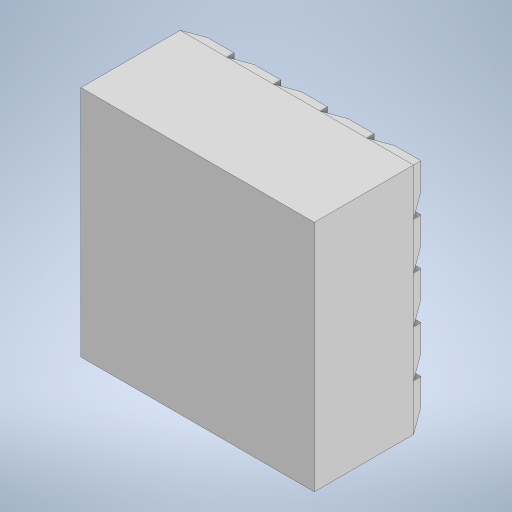
# Autodesk Inventor part: LI0013-FOOT
Saved by Autodesk Inventor 2023 (Build 270158000, 158)
## iProperties
Created: 2023-05-02
Part Number: LI0013-FOOT
Material: Generic
Document SubType Name: Modeling
Designer: Louis
Density: 1 g/cm^3
Appearance: Default
Author: Louis
Autodesk Inventor part; units mm, degrees
ref_plane "YZ Plane" through (0, 0, 0) normal (1, 0, 0) x (0, 1, 0)
ref_plane "XZ Plane" through (0, 0, 0) normal (0, 1, 0) x (-1, 0, 0)
ref_plane "XY Plane" through (0, 0, 0) normal (0, 0, 1) x (1, 0, 0)
sketch "Sketch1" plane through (0, 0, 0) normal (0, 0, 1) x (1, 0, 0)
  line L0 (-20, 20) -> (20, 20)
  line L1 (20, 20) -> (20, -20)
  line L2 (20, -20) -> (-20, -20)
  line L3 (-20, -20) -> (-20, 20)
  point P0 (0, 0)
  point P1 (-20, 0)
  point P2 (0, 20)
  dimension "d0" = 40
  dimension "d1" = 40
  constraints: 8 end point, 2 midpoint, 2 parallel, 1 horizontal, 1 horizontal alignment, 1 perpendicular, 1 vertical alignment
  measures "d0" distance of L0.start L0.end
  measures "d1" distance of L0.end L1.end
extrude "Extrusion1" add sketch "Sketch1" along normal blind 20
sketch "Sketch2" plane through (-20, -20, 0) normal (0, -1, 0) x (1, 0, 0)
  line L0 (0, 0) -> (40, 0) projected
  line L1 (0, 0) -> (0, 20) projected
  line L2 (40, 0) -> (0, 0)
  line L3 (0, 0) -> (0, 3)
  line L4 (0, 3) -> (40, 3)
  line L5 (40, 3) -> (40, 0)
  line L6 (40, 0) -> (0, 0) projected
  line L7 (32, 0) -> (32, 3)
  line L8 (32, 3) -> (33.7321, 0)
  line L9 (32, 3) -> (30.2679, 0)
  point P0 (20, 0)
  point P1 (40, 1.5)
  dimension "d4" = 3
  dimension "d5" = 8
  dimension "d6" = 30
  dimension "d7" = 30
  constraints: 14 end point, 5 point on line, 2 parallel, 2 perpendicular, 1 horizontal, 1 midpoint
  measures "d4" distance between parallel lines of L0 L4
  measures "d5" distance from line of point (40, 1.5) L7
  measures "d6" angle of L8 L7
  measures "d7" angle of L7 L9
extrude "Extrusion2" cut sketch "Sketch2" against normal through all contours L9 L7 L0 | L7 L8 L0
pattern_linear "Rectangular Pattern1" count 4 spacing 8 along (-1, 0, 0) of "Extrusion2"
ref_plane "Work Plane1" through (-20, 0, 20) normal (0, -1, 0) x (1, 0, 0)
ref_plane "Work Plane2" through (0, -20, 0) normal (1, 0, 0) x (0, 0, -1)
pattern_circular "Circular Pattern1" count 2 over 90 about axis through (0, 0, 20) along (0, 0, 1) of "Extrusion2", "Rectangular Pattern1"
chamfer "Chamfer1" distance 3 angle 30 5 edges at (16.866, 20, 0) (8, 20, 0) (0, 20, 0) (-8, 20, 0) (-16.866, 20, 0) measured on face at (-1.3333, 20, 14.3333)
chamfer "Chamfer2" distance 3 angle 30 5 edges at (-20, 16.0003, 0) (-20, 8, 0) (-20, 0, 0) (-20, -8, 0) (-20, -16.866, 0) measured on face at (-20, -1.3333, 14.3333)
chamfer "Chamfer3" distance 3 angle 30 5 edges at (-16.0003, -20, 0) (-8, -20, 0) (0, -20, 0) (8, -20, 0) (16.866, -20, 0) measured on face at (1.3333, -20, 14.3333)
chamfer "Chamfer4" distance 3 angle 30 5 edges at (20, -16.0003, 0) (20, -8, 0) (20, 8, 0) (20, 0, 0) (20, 16.0003, 0) measured on face at (20, 1.3333, 14.3333)
body "Solid1"
